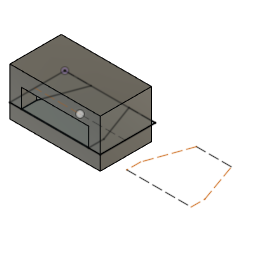
IR sensor mount V10 (Autodesk Fusion 360 design; units mm, degrees)
Autodesk Fusion 360 part; units mm, degrees
note: some values were not read from the file. Set by a fixed rule: which sketch regions a step uses.
sketch "Sketch1" plane through (0, 0, 0) normal (0, 0, 1) x (1, 0, 0)
  line L0 (0, 0) -> (25, 0)
  line L1 (25, 0) -> (25, -15.2)
  line L2 (25, -15.2) -> (0, -15.2)
  line L3 (0, -15.2) -> (0, 0)
  line L4 (7.25, 0) -> (3.2, -11)
  line L5 (17.75, 0) -> (21.8, -11)
  line L6 (3.2, -11) -> (3.2, -15.2)
  line L7 (21.8, -11) -> (21.8, -15.2)
  line L8 (3.2, -15.2) -> (21.8, -15.2) construction
  line L9 (12.5, -8.3) -> (25, -8.3) construction
  line L10 (12.5, -8.3) -> (0, -8.3) construction
  line L11 (0, 0) -> (7.25, 0) construction
  line L12 (17.75, 0) -> (25, 0) construction
  line L13 (36.4201, 0) -> (32.3701, -11.4) construction
  line L14 (32.3701, -11.4) -> (32.3701, -15.2) construction
  line L15 (32.3701, -15.2) -> (50.1701, -15.2) construction
  line L16 (50.1701, -15.2) -> (50.1701, -11.4) construction
  line L17 (50.1701, -11.4) -> (46.1201, 0) construction
  line L18 (36.4201, 0) -> (46.1201, 0) construction
  dimension "d1" = 25
  dimension "d2" = 15.2
  dimension "d3" = 10.5
  dimension "d5" = 18.6
  dimension "d10" = 11
  dimension "d14" = 8.3
  dimension "d26" = 3.8
  dimension "d27" = 17.8
  dimension "d28" = 9.7
  dimension "d29" = 15.2
  constraint horizontal L0
  constraint vertical L1
  constraint horizontal L2
  constraint vertical L3
  constraint coincident L0 L4.start
  constraint coincident L0 L5.start
  constraint perpendicular L0 L6
  constraint vertical L7
  constraint equal L6 L7
  constraint parallel L0 L8
  constraint coincident L0.start L3.end
  constraint equal L4 L5
  constraint coincident L2 L6.end
  constraint coincident L1 L9.end
  constraint perpendicular L1 L9
  constraint coincident L3 L10.end
  constraint perpendicular L3 L10
  constraint equal L9 L10
  constraint equal L11 L12
  constraint coincident L0 L13.start
  constraint perpendicular L10 L14
  constraint perpendicular L14 L15
  constraint perpendicular L9 L16
  constraint coincident L0 L17.end
  constraint equal L14 L16
  constraint equal L13 L17
  measures "d1" distance of L0.start L0.end
  measures "d2" distance of L0 L2
  measures "d3" distance of L4.start L5.start
  measures "d5" distance of L6.end L7.end
  measures "d10" distance of L0 L4.end
  measures "d14" distance of L0 L9.start
  measures "d26" distance of L13.end L14.end
  measures "d27" distance of L14.end L15.end
  measures "d28" distance of L13.start L17.end
  measures "d29" distance of L13.start L15
extrude "Extrude1" add sketch "Sketch1" against normal blind 4 makes body 1
extrude "Extrude2" add sketch "Sketch1" along normal blind 5.2 contours L0 L2 L3 L4 L6 | L0 L1 L2 L5 L7 bodies 1
extrude "Extrude3" add sketch "Sketch1" along normal blind 4 from surface at 5.2 separate body makes body 2
combine "Combine1" operation add target body 1 tool bodies 2
extrude "Extrude5" cut 1 faces at (22.5833, 0, 1.7333) along direction (0, -1, 0) blind 1 on bodies 1 bodies 1
fillet "Fillet2" radius 1 2 edges at (6.8818, -1, 2.6) (18.1182, -1, 2.6) on bodies 1
equation "d3 = 9.7 mm + 0.8 mm"
equation "d5 = 17.8 mm + 0.8 mm"
equation "d14 = 8.4 mm - 0.1 mm"
equation "d17 = 5 mm + 0.2 mm"
